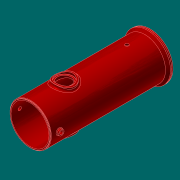
# Autodesk Inventor part: A1-19027-400-10 HCWI liner - trunk
Saved by Autodesk Inventor 2017.3 (Build 213256000, 256)
## iProperties
Created: 2019-08-16
Part Number: A1-19027-400-10 HCWI liner - trunk
Material: Iron, HCWI
Document SubType Name: Modeling
Designer: GVD
Density: 7.33517 g/cm^3
Appearance: Iron Gray(1)
Mass: 1.33384e+06 g
Surface Area: 112420 cm^2
Volume: 181841 cm^3
Author: GVD
Autodesk Inventor part; units mm, degrees
ref_plane "XY Plane" through (0, 0, 0) normal (0, 0, 1) x (1, 0, 0)
sketch "Sketch1" plane through (0, 0, 0) normal (0, 0, 1) x (1, 0, 0)
  circle A0 centre (0, 0) radius 361.95
  circle A1 centre (0, 0) radius 393.7
  dimension "d0" = 723.9
  dimension "d1" = 787.4
  constraints: 2 centre point, 2 coincident
  measures "d0" diameter of A0
  measures "d1" diameter of A1
extrude "Extrusion1" add sketch "Sketch1" along normal blind 2286
sketch "Sketch2" plane through (0, 0, 0) normal (0, 0, -1) x (-1, 0, 0)
  circle A0 centre (0, 0) radius 393.7 projected
  circle A1 centre (0, 0) radius 441.325
  dimension "d4" = 882.65
  constraints: 1 centre point, 1 coincident
  measures "d4" diameter of A1
extrude "Extrusion2" add sketch "Sketch2" against normal blind 50.8
sketch "Sketch3" plane through (0, 0, 0) normal (0, 0, -1) x (-1, 0, 0)
  circle A0 centre (0, 0) radius 441.325 projected
  circle A1 centre (0, 0) radius 437.896
  dimension "d7" = 875.792
  constraints: 1 centre point, 1 coincident
  measures "d7" diameter of A1
extrude "Extrusion3" cut sketch "Sketch3" against normal blind 25.4
chamfer "Chamfer1" distance 47.625 angle 45 1 edges at (-393.7, 0, 50.8)
sketch "Sketch4" plane through (0, 0, 2286) normal (0, 0, 1) x (1, 0, 0)
  circle A0 centre (0, 0) radius 393.7 projected
  circle A1 centre (0, 0) radius 380.746
  dimension "d13" = 761.492
  constraints: 1 centre point, 1 coincident
  measures "d13" diameter of A1
extrude "Extrusion4" cut sketch "Sketch4" against normal blind 12.7
chamfer "Chamfer2" distance 0.7937 angle 45 1 edges at (-380.746, 0, 2286)
fillet "Fillet1" radius 0.7937 2 edges at (-380.746, 0, 2273.3) (437.896, 0, 25.4)
sketch "Sketch5" plane through (0, 0, 0) normal (0, 1, 0) x (-1, 0, 0)
  circle A0 centre (0, 440) radius 33
  circle A1 centre (0, 1632) radius 133.35
  point P0 (0, 0)
  dimension "d20" = 66
  dimension "d21" = 440
  dimension "d22" = 266.7
  dimension "d23" = 1192
  constraints: 2 centre point, 2 vertical alignment
  measures "d20" diameter of A0
  measures "d21" distance of point (0, 0) A0.centre
  measures "d22" diameter of A1
  measures "d23" distance of A0.centre A1.centre
extrude "Extrusion5" cut sketch "Sketch5" along normal through all both and the other way through all
ref_plane "Work Plane1" through (-393.7, 0, 0) normal (-1, 0, 0) x (0, -1, 0)
sketch "Sketch6" plane through (-393.7, 0, 0) normal (-1, 0, 0) x (0, -1, 0)
  circle A0 centre (0, 2120) radius 50.8
  circle A1 centre (0, 2120) radius 31.75
  point P0 (0, 0)
  dimension "d26" = 101.6
  dimension "d27" = 63.5
  dimension "d28" = 2120
  constraints: 2 centre point, 1 coincident, 1 vertical alignment
  measures "d26" diameter of A0
  measures "d27" diameter of A1
  measures "d28" distance of A0.centre point (0, 0)
extrude "Extrusion6" cut sketch "Sketch6" against normal up to surface (393.7 mm away) contours A1
extrude "Extrusion7" add sketch "Sketch6" against normal up to surface round surface about axis through (0, 0, 0) along (0, 0, 1) radius 393.7 far side no
extrude "Extrusion8" add sketch "Sketch6" along normal blind 38.1
fillet "Fillet2" radius 12.7 3 edges at (-391.7862, -38.7723, 2152.823) (-391.7862, -38.7722, 2087.1768) (-390.4088, 50.8, 2120.0078)
pattern_circular "Circular Pattern1" count 2 over 360 about axis through (0, 0, -10) along (0, 0, 1) of "Extrusion6", "Extrusion7", "Extrusion8", "Fillet2"
ref_plane "Work Plane2" through (0, 393.7, 0) normal (0, 1, 0) x (-1, 0, 0)
sketch "Sketch7" plane through (0, 393.7, 0) normal (0, 1, 0) x (-1, 0, 0)
  circle A0 centre (0, 1632) radius 133.35 projected
  circle A1 centre (0, 1632) radius 190.5
  circle A2 centre (0, 1632) radius 161.925
  point P0 (0, 0)
  dimension "d39" = 381
  dimension "d42" = 323.85
  constraints: 2 centre point, 2 coincident
  measures "d39" diameter of A1
  measures "d42" diameter of A2
extrude "Extrusion9" add sketch "Sketch7" against normal up to surface contours A1 | A2 round surface about axis through (0, 0, 0) along (0, 0, 1) radius 393.7 far side no
sketch "Sketch8" plane through (0, 0, 0) normal (0, 0, 1) x (1, 0, 0)
  circle A0 centre (0, 0) radius 441.325
  dimension "d43" = 882.65
  constraints: 1 centre point, 1 coincident
  measures "d43" diameter of A0
surface extrude "ExtrusionSrf1" sketch "Sketch8" along normal blind 2286 shown no curves A0
extrude "Extrusion10" add sketch "Sketch7" along normal up to surface contours A1 round surface about axis through (0, 0, 0) along (0, 0, 1) radius 441.325 far side no
fillet "Fillet3" radius 44.45 3 edges at (-144.9514, 366.0448, 1755.6097) (-144.9518, 366.0446, 1508.3909) (190.5, 344.5424, 1632.1285)
fillet "Fillet4" radius 0.7937 1 edges at (161.925, 393.7, 1632)
pattern_circular "Circular Pattern2" count 2 over 360 about axis through (0, 0, -10) along (0, 0, 1) of "Extrusion9", "Extrusion10", "Fillet3", "Fillet4"
equation "\"d10\" = -0.5 * d1 + 0.5 * d4"
equation "\"d44\" = d2"
equation "\"d46\" = d2"
equation "\"d2\" = 2286"
body "Solid1"
body "Srf1"
